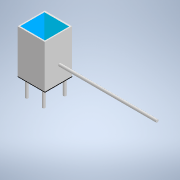
# Autodesk Inventor part: Water tank
Saved by Autodesk Inventor 2021 (Build 250183000, 183)
## iProperties
Created: 2021-07-14
Part Number: Water tank
Material: Generic
Document SubType Name: Modeling
Designer: shifa
Density: 1 g/cm^3
Appearance: Default
Author: shifa
Autodesk Inventor part; units mm, degrees
ref_plane "YZ Plane" through (0, 0, 0) normal (1, 0, 0) x (0, 1, 0)
ref_plane "XZ Plane" through (0, 0, 0) normal (0, 1, 0) x (-1, 0, 0)
ref_plane "XY Plane" through (0, 0, 0) normal (0, 0, 1) x (1, 0, 0)
sketch "Sketch1" plane through (0, 0, 0) normal (0, 1, 0) x (-1, 0, 0)
  line L0 (0, 0) -> (50, 0)
  line L1 (50, 0) -> (50, -50)
  line L2 (50, -50) -> (0, -50)
  line L3 (0, -50) -> (0, 0)
  circle A0 centre (37.6883, -4.8163) radius 2.5
  circle A1 centre (37.6883, -43.3405) radius 2.5
  circle A2 centre (6.6955, -43.3405) radius 2.5
  circle A3 centre (6.6955, -4.8163) radius 2.5
  dimension "d0" = 50
  dimension "d1" = 50
  dimension "d6" = 5
  dimension "d9" = 5
  dimension "d10" = 5
  dimension "d11" = 5
  dimension "d20" = 25.9928
  dimension "d21" = 38.5242
  constraints: 8 end point, 4 centre point, 2 parallel, 1 horizontal, 1 perpendicular
  measures "d0" distance of L1.end L2.end
  measures "d1" distance of L0.end L1.end
  measures "d6" diameter of A0
  measures "d9" diameter of A1
  measures "d10" diameter of A2
  measures "d11" diameter of A3
  measures "d21" distance of A2.centre A3.centre
extrude "Extrusion1" add sketch "Sketch1" along normal blind 80 contours L0 L1 L2 L3 | A0 | A1 | A2 | A3
sketch "Sketch2" plane through (0, 80, 0) normal (0, 1, 0) x (1, 0, 0)
  line L0 (-47.6071, 46.9807) -> (-2.1924, 46.9807)
  line L1 (-2.1924, 46.9807) -> (-2.1924, 2.5056)
  line L2 (-2.1924, 2.5056) -> (-47.6071, 2.5056)
  line L3 (-47.6071, 2.5056) -> (-47.6071, 46.9807)
  point P0 (0, 0)
  constraints: 8 end point, 2 parallel, 1 horizontal, 1 perpendicular
extrude "Extrusion2" cut sketch "Sketch2" against normal blind 48
extrude "Extrusion3" add sketch "Sketch1" against normal blind 30 contours A0 | A1 | A2 | A3
sketch "Sketch6" plane through (0, 0, 0) normal (1, 0, 0) x (0, 0, -1)
  circle A0 centre (27.1417, 30.3837) radius 2.5
  point P0 (0, 0)
  dimension "d22" = 5
  constraints: 1 centre point
  measures "d22" diameter of A0
extrude "Extrusion6" add sketch "Sketch6" along normal blind 180
body "Solid1"
